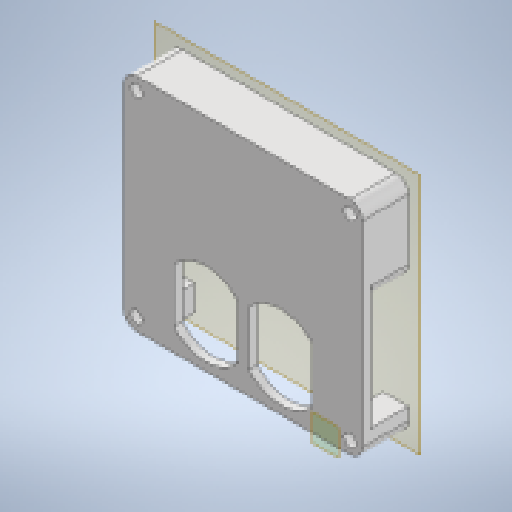
# Autodesk Inventor part: house_V6
Saved by Autodesk Inventor 2023 (Build 270158000, 158)
## iProperties
Created: 2023-03-15
Part Number: house_V6
Material: Generic
Document SubType Name: Modeling
Designer: shrey
Density: 1 g/cm^3
Appearance: Default
Author: shrey
Autodesk Inventor part; units mm, degrees
ref_plane "YZ Plane" through (0, 0, 0) normal (1, 0, 0) x (0, 1, 0)
ref_plane "XZ Plane" through (0, 0, 0) normal (0, 1, 0) x (-1, 0, 0)
ref_plane "Work Plane1" through (-29.0856, 4.4467, 21.749) normal (0, 0, 1) x (1, 0, 0)
ref_plane "Work Plane2" through (-5, -17, 36.649) normal (0, 0, -1) x (1, 0, 0)
ref_plane "Work Plane3" through (-40.5939, -3, 26.249) normal (0, 0, -1) x (0, 1, 0)
sketch "Sketch1" plane through (-29.0856, 4.4467, 21.749) normal (0, 0, 1) x (1, 0, 0)
  arc A0 (29.0856, 24.0967) -> (26.5856, 26.5967) centre (26.5856, 24.0967) ccw projected
  line L0 (26.5856, 26.5967) -> (-25.6023, 26.5967) projected
  arc A1 (-25.6023, 26.5967) -> (-28.1023, 24.0967) centre (-25.6023, 24.0967) ccw projected
  line L1 (-28.1023, 24.0967) -> (-28.1023, -23.9467) projected
  arc A2 (-28.1023, -23.9467) -> (-25.6023, -26.4467) centre (-25.6023, -23.9467) ccw projected
  line L2 (-25.6023, -26.4467) -> (26.5856, -26.4467) projected
  line L3 (29.0856, -23.9467) -> (29.0856, 24.0967)
  circle A3 centre (26.0856, -23.4467) radius 1.45 construction
  line L4 (0.4916, -38.3665) -> (0.4916, 43.9409) construction
  line L5 (29.0856, 26.5967) -> (-28.1023, 26.5967)
  line L6 (-28.1023, 26.5967) -> (-28.1023, 6.0209)
  line L7 (-28.1023, 6.0209) -> (29.0856, 6.0209)
  line L8 (29.0856, 6.0209) -> (29.0856, 26.5967)
  line L9 (30.8116, -0.0755) -> (30.8114, -0.0755)
  line L10 (29.0856, -23.9467) -> (29.0856, -26.4467)
  line L11 (29.0856, -26.4467) -> (26.5856, -26.4467)
  line L12 (-25.6023, -26.4467) -> (-28.1023, -26.4467)
  line L13 (-28.1023, -26.4467) -> (-28.1023, -23.9467)
  circle A4 centre (26.0856, -23.4467) radius 3 construction
  circle A5 centre (26.0856, -23.4467) radius 1.45
  circle A6 centre (-25.1024, -23.4467) radius 1.45 construction
  circle A7 centre (-25.1024, -23.4467) radius 1.45
  circle A8 centre (26.0856, 23.5963) radius 1.45 construction
  circle A9 centre (26.0856, 23.5963) radius 1.45
  circle A10 centre (-25.1024, 23.5963) radius 1.45 construction
  circle A11 centre (-25.1024, 23.5963) radius 1.45
  line L14 (29.0856, -26.4467) -> (23.0856, -26.4467)
  line L15 (23.0856, -26.4467) -> (23.0856, -20.4467)
  line L16 (23.0856, -20.4467) -> (29.0856, -20.4467)
  line L17 (29.0856, -20.4467) -> (29.0856, -26.4467)
  line L18 (-28.1023, -26.4467) -> (-22.1023, -26.4467)
  line L19 (-22.1023, -26.4467) -> (-22.1023, -20.4467)
  line L20 (-22.1023, -20.4467) -> (-28.1023, -20.4467)
  line L21 (-28.1023, -20.4467) -> (-28.1023, -26.4467)
  spline S0 degree 3 poles (31.7798, -5.9724) (31.66, -5.7823) (31.4802, -5.4972) (31.2591, -5.1058) (31.1003, -4.8085) (30.9498, -4.5069) (30.8081, -4.201) (30.6761, -3.8909) (30.5547, -3.5764) (30.4456, -3.2574) (30.3497, -2.9341) (30.2872, -2.6602) (30.2421, -2.4401) (30.1945, -2.2782) (30.1301, -2.1222) (30.0461, -1.9754) (29.9577, -1.8658) (29.8777, -1.7866) (29.8102, -1.7361) (29.741, -1.6877) (29.6647, -1.6516) (29.5872, -1.6181) (29.5051, -1.5983) (29.4223, -1.5815) (29.3098, -1.5775) (29.1694, -1.5801) (29.0291, -1.5775) (28.9165, -1.5815) (28.8338, -1.5983) (28.7517, -1.6181) (28.6742, -1.6516) (28.5979, -1.6877) (28.5287, -1.7361) (28.4611, -1.7866) (28.3812, -1.8658) (28.2927, -1.9754) (28.2088, -2.1222) (28.1444, -2.2782) (28.0967, -2.4401) (28.0516, -2.6602) (27.9892, -2.9341) (27.8932, -3.2574) (27.7842, -3.5764) (27.6628, -3.8909) (27.5307, -4.201) (27.389, -4.5069) (27.2385, -4.8085) (27.0797, -5.1058) (26.8587, -5.4972) (26.6789, -5.7823) (26.559, -5.9724) knots -1.0784 -1.0784 -1.0784 -1.0784 -1.010995 -0.977291 -0.943586 -0.909882 -0.876178 -0.842474 -0.80877 -0.775067 -0.741365 -0.707665 -0.690816 -0.67397 -0.657123 -0.640284 -0.623449 -0.615023 -0.606598 -0.598176 -0.589749 -0.581327 -0.572901 -0.564477 -0.556053 -0.5392 -0.522347 -0.513923 -0.505499 -0.497074 -0.488651 -0.480225 -0.471802 -0.463377 -0.454951 -0.438116 -0.421277 -0.40443 -0.387584 -0.370735 -0.337035 -0.303333 -0.26963 -0.235926 -0.202222 -0.168518 -0.134814 -0.101109 -0.067405 0 0 0 0 construction
  line L22 (26.559, -5.9724) -> (25.4968, -5.9724) construction
  spline S1 degree 3 poles (25.4968, -5.9724) (25.377, -5.7823) (25.1972, -5.4972) (24.9761, -5.1058) (24.8173, -4.8085) (24.6668, -4.5069) (24.5251, -4.201) (24.3931, -3.8909) (24.2717, -3.5764) (24.1626, -3.2574) (24.0667, -2.9341) (24.0042, -2.6602) (23.9591, -2.4401) (23.9115, -2.2782) (23.8471, -2.1222) (23.7631, -1.9754) (23.6747, -1.8658) (23.5947, -1.7866) (23.5272, -1.7361) (23.458, -1.6877) (23.3817, -1.6516) (23.3042, -1.6181) (23.2221, -1.5983) (23.1393, -1.5815) (23.0268, -1.5775) (22.8864, -1.5801) (22.7461, -1.5775) (22.6335, -1.5815) (22.5508, -1.5983) (22.4687, -1.6181) (22.3912, -1.6516) (22.3149, -1.6877) (22.2457, -1.7361) (22.1781, -1.7866) (22.0982, -1.8658) (22.0097, -1.9754) (21.9258, -2.1222) (21.8614, -2.2782) (21.8137, -2.4401) (21.7686, -2.6602) (21.7062, -2.9341) (21.6102, -3.2574) (21.5012, -3.5764) (21.3798, -3.8909) (21.2477, -4.201) (21.106, -4.5069) (20.9555, -4.8085) (20.7967, -5.1058) (20.5757, -5.4972) (20.3959, -5.7823) (20.276, -5.9724) knots -1.0784 -1.0784 -1.0784 -1.0784 -1.010995 -0.977291 -0.943586 -0.909882 -0.876178 -0.842474 -0.80877 -0.775067 -0.741365 -0.707665 -0.690816 -0.67397 -0.657123 -0.640284 -0.623449 -0.615023 -0.606598 -0.598176 -0.589749 -0.581327 -0.572901 -0.564477 -0.556053 -0.5392 -0.522347 -0.513923 -0.505499 -0.497074 -0.488651 -0.480225 -0.471802 -0.463377 -0.454951 -0.438116 -0.421277 -0.40443 -0.387584 -0.370735 -0.337035 -0.303333 -0.26963 -0.235926 -0.202222 -0.168518 -0.134814 -0.101109 -0.067405 0 0 0 0 construction
  line L23 (20.276, -5.9724) -> (19.2138, -5.9724) construction
  spline S2 degree 3 poles (19.2138, -5.9724) (19.094, -5.7823) (18.9142, -5.4972) (18.6931, -5.1058) (18.5343, -4.8085) (18.3838, -4.5069) (18.2421, -4.201) (18.1101, -3.8909) (17.9887, -3.5764) (17.8796, -3.2574) (17.7837, -2.9341) (17.7212, -2.6602) (17.6761, -2.4401) (17.6285, -2.2782) (17.5641, -2.1222) (17.4801, -1.9754) (17.3917, -1.8658) (17.3117, -1.7866) (17.2442, -1.7361) (17.175, -1.6877) (17.0987, -1.6516) (17.0212, -1.6181) (16.9391, -1.5983) (16.8563, -1.5815) (16.7438, -1.5775) (16.6034, -1.5801) (16.4631, -1.5775) (16.3505, -1.5815) (16.2678, -1.5983) (16.1857, -1.6181) (16.1082, -1.6516) (16.0319, -1.6877) (15.9627, -1.7361) (15.8951, -1.7866) (15.8152, -1.8658) (15.7267, -1.9754) (15.6428, -2.1222) (15.5784, -2.2782) (15.5307, -2.4401) (15.4856, -2.6602) (15.4232, -2.9341) (15.3272, -3.2574) (15.2182, -3.5764) (15.0968, -3.8909) (14.9647, -4.201) (14.823, -4.5069) (14.6725, -4.8085) (14.5137, -5.1058) (14.2927, -5.4972) (14.1129, -5.7823) (13.993, -5.9724) knots -1.0784 -1.0784 -1.0784 -1.0784 -1.010995 -0.977291 -0.943586 -0.909882 -0.876178 -0.842474 -0.80877 -0.775067 -0.741365 -0.707665 -0.690816 -0.67397 -0.657123 -0.640284 -0.623449 -0.615023 -0.606598 -0.598176 -0.589749 -0.581327 -0.572901 -0.564477 -0.556053 -0.5392 -0.522347 -0.513923 -0.505499 -0.497074 -0.488651 -0.480225 -0.471802 -0.463377 -0.454951 -0.438116 -0.421277 -0.40443 -0.387584 -0.370735 -0.337035 -0.303333 -0.26963 -0.235926 -0.202222 -0.168518 -0.134814 -0.101109 -0.067405 0 0 0 0 construction
  line L24 (13.993, -5.9724) -> (12.9308, -5.9724) construction
  spline S3 degree 3 poles (12.9308, -5.9724) (12.811, -5.7823) (12.6312, -5.4972) (12.4101, -5.1058) (12.2513, -4.8085) (12.1008, -4.5069) (11.9591, -4.201) (11.8271, -3.8909) (11.7057, -3.5764) (11.5966, -3.2574) (11.5007, -2.9341) (11.4382, -2.6602) (11.3931, -2.4401) (11.3455, -2.2782) (11.2811, -2.1222) (11.1971, -1.9754) (11.1087, -1.8658) (11.0287, -1.7866) (10.9612, -1.7361) (10.892, -1.6877) (10.8157, -1.6516) (10.7382, -1.6181) (10.6561, -1.5983) (10.5733, -1.5815) (10.4608, -1.5775) (10.3204, -1.5801) (10.1801, -1.5775) (10.0675, -1.5815) (9.9848, -1.5983) (9.9027, -1.6181) (9.8252, -1.6516) (9.7489, -1.6877) (9.6797, -1.7361) (9.6121, -1.7866) (9.5322, -1.8658) (9.4437, -1.9754) (9.3598, -2.1222) (9.2954, -2.2782) (9.2477, -2.4401) (9.2026, -2.6602) (9.1402, -2.9341) (9.0442, -3.2574) (8.9352, -3.5764) (8.8138, -3.8909) (8.6817, -4.201) (8.54, -4.5069) (8.3895, -4.8085) (8.2307, -5.1058) (8.0097, -5.4972) (7.8299, -5.7823) (7.71, -5.9724) knots -1.0784 -1.0784 -1.0784 -1.0784 -1.010995 -0.977291 -0.943586 -0.909882 -0.876178 -0.842474 -0.80877 -0.775067 -0.741365 -0.707665 -0.690816 -0.67397 -0.657123 -0.640284 -0.623449 -0.615023 -0.606598 -0.598176 -0.589749 -0.581327 -0.572901 -0.564477 -0.556053 -0.5392 -0.522347 -0.513923 -0.505499 -0.497074 -0.488651 -0.480225 -0.471802 -0.463377 -0.454951 -0.438116 -0.421277 -0.40443 -0.387584 -0.370735 -0.337035 -0.303333 -0.26963 -0.235926 -0.202222 -0.168518 -0.134814 -0.101109 -0.067405 0 0 0 0 construction
  line L25 (7.71, -5.9724) -> (6.6478, -5.9724) construction
  spline S4 degree 3 poles (6.6478, -5.9724) (6.528, -5.7823) (6.3482, -5.4972) (6.1271, -5.1058) (5.9683, -4.8085) (5.8178, -4.5069) (5.6761, -4.201) (5.5441, -3.8909) (5.4227, -3.5764) (5.3136, -3.2574) (5.2177, -2.9341) (5.1552, -2.6602) (5.1101, -2.4401) (5.0625, -2.2782) (4.9981, -2.1222) (4.9141, -1.9754) (4.8257, -1.8658) (4.7457, -1.7866) (4.6782, -1.7361) (4.609, -1.6877) (4.5327, -1.6516) (4.4552, -1.6181) (4.3731, -1.5983) (4.2903, -1.5815) (4.1778, -1.5775) (4.0374, -1.5801) (3.8971, -1.5775) (3.7845, -1.5815) (3.7018, -1.5983) (3.6197, -1.6181) (3.5422, -1.6516) (3.4659, -1.6877) (3.3967, -1.7361) (3.3291, -1.7866) (3.2492, -1.8658) (3.1607, -1.9754) (3.0768, -2.1222) (3.0124, -2.2782) (2.9647, -2.4401) (2.9196, -2.6602) (2.8572, -2.9341) (2.7612, -3.2574) (2.6522, -3.5764) (2.5308, -3.8909) (2.3987, -4.201) (2.257, -4.5069) (2.1065, -4.8085) (1.9477, -5.1058) (1.7267, -5.4972) (1.5469, -5.7823) (1.427, -5.9724) knots -1.0784 -1.0784 -1.0784 -1.0784 -1.010995 -0.977291 -0.943586 -0.909882 -0.876178 -0.842474 -0.80877 -0.775067 -0.741365 -0.707665 -0.690816 -0.67397 -0.657123 -0.640284 -0.623449 -0.615023 -0.606598 -0.598176 -0.589749 -0.581327 -0.572901 -0.564477 -0.556053 -0.5392 -0.522347 -0.513923 -0.505499 -0.497074 -0.488651 -0.480225 -0.471802 -0.463377 -0.454951 -0.438116 -0.421277 -0.40443 -0.387584 -0.370735 -0.337035 -0.303333 -0.26963 -0.235926 -0.202222 -0.168518 -0.134814 -0.101109 -0.067405 0 0 0 0 construction
  line L26 (1.427, -5.9724) -> (0.3648, -5.9724) construction
  spline S5 degree 3 poles (0.3648, -5.9724) (0.245, -5.7823) (0.0652, -5.4972) (-0.1559, -5.1058) (-0.3147, -4.8085) (-0.4652, -4.5069) (-0.6069, -4.201) (-0.7389, -3.8909) (-0.8603, -3.5764) (-0.9694, -3.2574) (-1.0653, -2.9341) (-1.1278, -2.6602) (-1.1729, -2.4401) (-1.2205, -2.2782) (-1.2849, -2.1222) (-1.3689, -1.9754) (-1.4573, -1.8658) (-1.5373, -1.7866) (-1.6048, -1.7361) (-1.674, -1.6877) (-1.7503, -1.6516) (-1.8278, -1.6181) (-1.9099, -1.5983) (-1.9927, -1.5815) (-2.1052, -1.5775) (-2.2456, -1.5801) (-2.3859, -1.5775) (-2.4985, -1.5815) (-2.5812, -1.5983) (-2.6633, -1.6181) (-2.7408, -1.6516) (-2.8171, -1.6877) (-2.8863, -1.7361) (-2.9539, -1.7866) (-3.0338, -1.8658) (-3.1223, -1.9754) (-3.2062, -2.1222) (-3.2706, -2.2782) (-3.3183, -2.4401) (-3.3634, -2.6602) (-3.4258, -2.9341) (-3.5218, -3.2574) (-3.6308, -3.5764) (-3.7522, -3.8909) (-3.8843, -4.201) (-4.026, -4.5069) (-4.1765, -4.8085) (-4.3353, -5.1058) (-4.5563, -5.4972) (-4.7361, -5.7823) (-4.856, -5.9724) knots -1.0784 -1.0784 -1.0784 -1.0784 -1.010995 -0.977291 -0.943586 -0.909882 -0.876178 -0.842474 -0.80877 -0.775067 -0.741365 -0.707665 -0.690816 -0.67397 -0.657123 -0.640284 -0.623449 -0.615023 -0.606598 -0.598176 -0.589749 -0.581327 -0.572901 -0.564477 -0.556053 -0.5392 -0.522347 -0.513923 -0.505499 -0.497074 -0.488651 -0.480225 -0.471802 -0.463377 -0.454951 -0.438116 -0.421277 -0.40443 -0.387584 -0.370735 -0.337035 -0.303333 -0.26963 -0.235926 -0.202222 -0.168518 -0.134814 -0.101109 -0.067405 0 0 0 0 construction
  line L27 (-4.856, -5.9724) -> (-5.9182, -5.9724) construction
  spline S6 degree 3 poles (-5.9182, -5.9724) (-6.038, -5.7823) (-6.2178, -5.4972) (-6.4389, -5.1058) (-6.5977, -4.8085) (-6.7482, -4.5069) (-6.8899, -4.201) (-7.0219, -3.8909) (-7.1433, -3.5764) (-7.2524, -3.2574) (-7.3483, -2.9341) (-7.4108, -2.6602) (-7.4559, -2.4401) (-7.5035, -2.2782) (-7.5679, -2.1222) (-7.6519, -1.9754) (-7.7403, -1.8658) (-7.8203, -1.7866) (-7.8878, -1.7361) (-7.957, -1.6877) (-8.0333, -1.6516) (-8.1108, -1.6181) (-8.1929, -1.5983) (-8.2757, -1.5815) (-8.3882, -1.5775) (-8.5286, -1.5801) (-8.6689, -1.5775) (-8.7815, -1.5815) (-8.8642, -1.5983) (-8.9463, -1.6181) (-9.0238, -1.6516) (-9.1001, -1.6877) (-9.1693, -1.7361) (-9.2369, -1.7866) (-9.3168, -1.8658) (-9.4053, -1.9754) (-9.4892, -2.1222) (-9.5536, -2.2782) (-9.6013, -2.4401) (-9.6464, -2.6602) (-9.7088, -2.9341) (-9.8048, -3.2574) (-9.9138, -3.5764) (-10.0352, -3.8909) (-10.1673, -4.201) (-10.309, -4.5069) (-10.4595, -4.8085) (-10.6183, -5.1058) (-10.8393, -5.4972) (-11.0191, -5.7823) (-11.139, -5.9724) knots -1.0784 -1.0784 -1.0784 -1.0784 -1.010995 -0.977291 -0.943586 -0.909882 -0.876178 -0.842474 -0.80877 -0.775067 -0.741365 -0.707665 -0.690816 -0.67397 -0.657123 -0.640284 -0.623449 -0.615023 -0.606598 -0.598176 -0.589749 -0.581327 -0.572901 -0.564477 -0.556053 -0.5392 -0.522347 -0.513923 -0.505499 -0.497074 -0.488651 -0.480225 -0.471802 -0.463377 -0.454951 -0.438116 -0.421277 -0.40443 -0.387584 -0.370735 -0.337035 -0.303333 -0.26963 -0.235926 -0.202222 -0.168518 -0.134814 -0.101109 -0.067405 0 0 0 0 construction
  line L28 (-11.139, -5.9724) -> (-12.2012, -5.9724) construction
  spline S7 degree 3 poles (-12.2012, -5.9724) (-12.321, -5.7823) (-12.5008, -5.4972) (-12.7219, -5.1058) (-12.8807, -4.8085) (-13.0312, -4.5069) (-13.1729, -4.201) (-13.3049, -3.8909) (-13.4263, -3.5764) (-13.5354, -3.2574) (-13.6313, -2.9341) (-13.6938, -2.6602) (-13.7389, -2.4401) (-13.7865, -2.2782) (-13.8509, -2.1222) (-13.9349, -1.9754) (-14.0233, -1.8658) (-14.1033, -1.7866) (-14.1708, -1.7361) (-14.24, -1.6877) (-14.3163, -1.6516) (-14.3938, -1.6181) (-14.4759, -1.5983) (-14.5587, -1.5815) (-14.6712, -1.5775) (-14.8116, -1.5801) (-14.9519, -1.5775) (-15.0645, -1.5815) (-15.1472, -1.5983) (-15.2293, -1.6181) (-15.3068, -1.6516) (-15.3831, -1.6877) (-15.4523, -1.7361) (-15.5199, -1.7866) (-15.5998, -1.8658) (-15.6883, -1.9754) (-15.7722, -2.1222) (-15.8366, -2.2782) (-15.8843, -2.4401) (-15.9294, -2.6602) (-15.9918, -2.9341) (-16.0878, -3.2574) (-16.1968, -3.5764) (-16.3182, -3.8909) (-16.4503, -4.201) (-16.592, -4.5069) (-16.7425, -4.8085) (-16.9013, -5.1058) (-17.1223, -5.4972) (-17.3021, -5.7823) (-17.422, -5.9724) knots -1.0784 -1.0784 -1.0784 -1.0784 -1.010995 -0.977291 -0.943586 -0.909882 -0.876178 -0.842474 -0.80877 -0.775067 -0.741365 -0.707665 -0.690816 -0.67397 -0.657123 -0.640284 -0.623449 -0.615023 -0.606598 -0.598176 -0.589749 -0.581327 -0.572901 -0.564477 -0.556053 -0.5392 -0.522347 -0.513923 -0.505499 -0.497074 -0.488651 -0.480225 -0.471802 -0.463377 -0.454951 -0.438116 -0.421277 -0.40443 -0.387584 -0.370735 -0.337035 -0.303333 -0.26963 -0.235926 -0.202222 -0.168518 -0.134814 -0.101109 -0.067405 0 0 0 0 construction
  line L29 (-17.422, -5.9724) -> (-18.4842, -5.9724) construction
  spline S8 degree 3 poles (-18.4842, -5.9724) (-18.604, -5.7823) (-18.7838, -5.4972) (-19.0049, -5.1058) (-19.1637, -4.8085) (-19.3142, -4.5069) (-19.4559, -4.201) (-19.5879, -3.8909) (-19.7093, -3.5764) (-19.8184, -3.2574) (-19.9143, -2.9341) (-19.9768, -2.6602) (-20.0219, -2.4401) (-20.0695, -2.2782) (-20.1339, -2.1222) (-20.2179, -1.9754) (-20.3063, -1.8658) (-20.3863, -1.7866) (-20.4538, -1.7361) (-20.523, -1.6877) (-20.5993, -1.6516) (-20.6768, -1.6181) (-20.7589, -1.5983) (-20.8417, -1.5815) (-20.9542, -1.5775) (-21.0946, -1.5801) (-21.2349, -1.5775) (-21.3475, -1.5815) (-21.4302, -1.5983) (-21.5123, -1.6181) (-21.5898, -1.6516) (-21.6661, -1.6877) (-21.7353, -1.7361) (-21.8029, -1.7866) (-21.8828, -1.8658) (-21.9713, -1.9754) (-22.0552, -2.1222) (-22.1196, -2.2782) (-22.1673, -2.4401) (-22.2124, -2.6602) (-22.2748, -2.9341) (-22.3708, -3.2574) (-22.4798, -3.5764) (-22.6012, -3.8909) (-22.7333, -4.201) (-22.875, -4.5069) (-23.0255, -4.8085) (-23.1843, -5.1058) (-23.4053, -5.4972) (-23.5851, -5.7823) (-23.705, -5.9724) knots -1.0784 -1.0784 -1.0784 -1.0784 -1.010995 -0.977291 -0.943586 -0.909882 -0.876178 -0.842474 -0.80877 -0.775067 -0.741365 -0.707665 -0.690816 -0.67397 -0.657123 -0.640284 -0.623449 -0.615023 -0.606598 -0.598176 -0.589749 -0.581327 -0.572901 -0.564477 -0.556053 -0.5392 -0.522347 -0.513923 -0.505499 -0.497074 -0.488651 -0.480225 -0.471802 -0.463377 -0.454951 -0.438116 -0.421277 -0.40443 -0.387584 -0.370735 -0.337035 -0.303333 -0.26963 -0.235926 -0.202222 -0.168518 -0.134814 -0.101109 -0.067405 0 0 0 0 construction
  line L30 (-23.705, -5.9724) -> (-24.7672, -5.9724) construction
  spline S9 degree 3 poles (-24.7672, -5.9724) (-25.0203, -5.5709) (-25.5973, -4.6557) (-26.3217, -2.6647) (-26.2743, -2.3174) (-26.6017, -1.8348) (-26.7085, -1.7546) (-26.812, -1.685) (-26.9085, -1.6251) (-27.2021, -1.5665) (-27.3381, -1.5791) (-27.5882, -1.5782) (-27.6989, -1.5807) (-27.923, -1.671) (-28.0168, -1.7314) (-28.1559, -1.8474) (-28.2174, -1.9297) (-28.3263, -2.0881) (-28.3821, -2.216) (-28.4787, -2.5326) (-28.4942, -2.6936) (-28.9709, -4.4107) (-29.8122, -5.6937) (-29.988, -5.9724) knots 0 0 0 0 0.142394 0.142394 0.262557 0.262557 0.314666 0.314666 0.34653 0.34653 0.372217 0.372217 0.394622 0.394622 0.411062 0.411062 0.432958 0.432958 0.48678 0.48678 0.562983 0.562983 0.900876 0.900876 0.900876 0.900876 construction
  line L31 (-29.988, -5.9724) -> (-29.988, 5.9209) construction
  line L32 (-29.988, 5.9209) -> (31.78, 5.9209) construction
  line L33 (31.78, 5.9209) -> (31.78, -5.9724) construction
  line L34 (31.78, -5.9724) -> (31.7798, -5.9724) construction
  point P0 (19.0856, -26.4467)
  point P1 (29.0856, -16.4467)
  point P2 (-28.1023, 6.0209)
  point P3 (29.0856, 6.0209)
  point P4 (-28.1023, -20.4467)
  point P5 (-25.6023, -26.4467)
  point P6 (-22.1023, -26.4467)
  point P7 (-25.6023, 26.5967)
  point P8 (-28.1023, 24.0967)
  point P9 (23.0856, -26.4467)
  point P10 (-28.1023, 24.0967)
  point P11 (-25.6023, 26.5967)
  point P12 (-28.1023, 6.0209)
  point P13 (29.0856, 6.0209)
  dimension "d56" = 0
  dimension "d68" = 3
  dimension "d69" = 3
  dimension "d72" = 51.188
  dimension "d75" = 47.043
  dimension "d93" = 0.1
  constraints: 38 end point, 9 centre point, 4 horizontal, 4 parallel, 3 perpendicular, 3 symmetric about line, 3 vertical, 2 coincident, 2 point on line, 2 tangent, 1 collinear, 1 concentric, 1 point on circle, 12 other
  measures "d56" distance between parallel lines of L1 L6
  measures "d68" distance from line of L2 A3.centre
  measures "d69" distance from line of A3.centre L3
  measures "d72" distance of A3.centre A6.centre
  measures "d75" distance of A3.centre A8.centre
  measures "d93" distance between parallel lines of L32 L7
extrude "Extrusion1" add sketch "Sketch1" along normal blind 9 contours L3 L7 L1 A1 L0 A0 | A0 L5 L8 | A1 L6 L5 | L3 L10 L11 L2 L15 L16 | L20 L19 L2 A2 L1 | A2 L12 L13
sketch "Sketch4" plane through (-29.0856, 4.4467, 30.749) normal (0, 0, 1) x (1, 0, 0)
  line L0 (-28.1023, -26.4467) -> (29.0856, -26.4467) projected
  line L1 (29.0856, 26.5967) -> (-28.1023, 26.5967) projected
  line L2 (29.0856, -26.4467) -> (-28.1023, -26.4467)
  line L3 (-28.1023, -26.4467) -> (-28.1023, 26.5967)
  line L4 (-28.1023, 26.5967) -> (29.0856, 26.5967)
  line L5 (29.0856, 26.5967) -> (29.0856, -26.4467)
  line L6 (0.4916, -26.4467) -> (0.4916, 26.5967) construction
  line L7 (11.9917, 4.4209) -> (6.9917, 4.4209)
  line L8 (6.9917, 4.4209) -> (6.9917, -0.0791)
  line L9 (6.9917, -0.0791) -> (11.9917, -0.0791)
  line L10 (11.9917, -0.0791) -> (11.9917, 4.4209)
  line L11 (11.9917, 4.4209) -> (6.9917, -0.0791) construction
  line L12 (6.9917, 4.4209) -> (11.9917, -0.0791) construction
  line L13 (-11.0084, 4.4209) -> (-6.0084, 4.4209)
  line L14 (-6.0084, 4.4209) -> (-6.0084, -0.0791)
  line L15 (-6.0084, -0.0791) -> (-11.0084, -0.0791)
  line L16 (-11.0084, -0.0791) -> (-11.0084, 4.4209)
  circle A0 centre (26.0856, 23.5963) radius 1.45 projected
  circle A1 centre (26.0856, -23.4467) radius 1.45 projected
  circle A2 centre (-25.1024, -23.4467) radius 1.45 projected
  circle A3 centre (-25.1024, 23.5963) radius 1.45 projected
  line L17 (29.78, 4.9209) -> (29.78, -0.5791) construction
  line L18 (-27.988, 4.9209) -> (29.78, 4.9209) construction
  line L19 (-27.988, -0.5791) -> (-27.988, 4.9209) construction
  line L20 (29.78, -0.5791) -> (-27.988, -0.5791) construction
  arc A4 (16.9917, -7.9467) -> (1.9917, -7.9467) centre (9.4917, -14.5611) ccw construction
  line L21 (1.9917, -20.9467) -> (1.9917, -7.9467) construction
  arc A5 (1.9917, -20.9467) -> (16.9917, -20.9467) centre (9.4917, -14.3323) ccw construction
  line L22 (16.9917, -7.9467) -> (16.9917, -20.9467) construction
  arc A6 (-16.0083, -20.9467) -> (-1.0083, -20.9467) centre (-8.5083, -14.3323) ccw construction
  line L23 (-1.0083, -7.9467) -> (-1.0083, -20.9467) construction
  arc A7 (-1.0083, -7.9467) -> (-16.0083, -7.9467) centre (-8.5083, -14.5611) ccw construction
  line L24 (-16.0083, -20.9467) -> (-16.0083, -7.9467) construction
  arc A8 (1.8917, -20.9844) -> (17.0917, -20.9844) centre (9.4917, -14.3323) ccw
  line L25 (1.8917, -20.9844) -> (1.8917, -7.909)
  arc A9 (17.0917, -7.909) -> (1.8917, -7.909) centre (9.4917, -14.5611) ccw
  line L26 (17.0917, -7.909) -> (17.0917, -20.9844)
  arc A10 (-16.1083, -20.9844) -> (-0.9083, -20.9844) centre (-8.5083, -14.3323) ccw
  line L27 (-16.1083, -20.9844) -> (-16.1083, -7.909)
  arc A11 (-0.9083, -7.909) -> (-16.1083, -7.909) centre (-8.5083, -14.5611) ccw
  line L28 (-0.9083, -7.909) -> (-0.9083, -20.9844)
  point P0 (29.0856, -4.4467)
  point P1 (23.0856, -26.4467)
  point P2 (9.4917, 2.1709)
  point P3 (23.0856, -26.4467)
  dimension "d84" = 5
  dimension "d94" = 0.5
  dimension "d96" = 0.5
  dimension "d97" = 0.1
  dimension "d98" = 0.1
  dimension "d99" = 0
  constraints: 38 end point, 8 point on circle, 4 centre point, 4 midpoint, 4 parallel, 4 symmetric about line, 2 horizontal, 2 perpendicular, 6 other
  measures "d84" distance between parallel lines of L10 L8
  measures "d94" distance between parallel lines of L20 L9
  measures "d96" distance between parallel lines of L18 L7
  measures "d97" radial gap between concentric circles of A5 A8
  measures "d98" radial gap between concentric circles of A6 A10
  measures "d99" horizontal distance of A5.centre point (9.492, 2.171)
extrude "Extrusion6" add sketch "Sketch4" along normal blind 2 contours L3 L1 L5 L0 | L10 L9 L8 L7 | L13 L14 L15 L16
extrude "Extrusion7" add sketch "Sketch4" against normal blind 2 contours L10 L9 L8 L7 | L13 L14 L15 L16
fillet "Fillet2" radius 3 6 edges at (0, -22, 27.249) (-57.1879, -22, 27.249) (0, 31.0434, 27.249) (-57.1879, 31.0434, 27.249) (0, 10.4676, 26.249) (-57.1879, 10.4676, 26.249)
body "Solid1"
